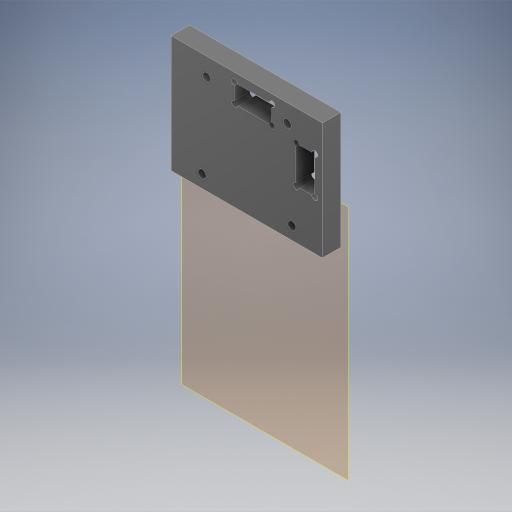
# Autodesk Inventor part: battery sideplate
Saved by Autodesk Inventor 2024 (Build 280153000, 153)
## iProperties
Created: 2024-09-04
Part Number: battery sideplate
Material: PMMA 플라스틱
Document SubType Name: Modeling
Designer: msi
Density: 1.188 g/cm^3
Appearance: 매끄러움 - 검은색
Author: msi
Autodesk Inventor part; units mm, degrees
ref_plane "YZ Plane" through (0, 0, 0) normal (1, 0, 0) x (0, 1, 0)
ref_plane "XZ Plane" through (0, 0, 0) normal (0, 1, 0) x (-1, 0, 0)
ref_plane "XY Plane" through (0, 0, 0) normal (0, 0, 1) x (1, 0, 0)
ref_plane "작업 평면1" through (0, 0, 0) normal (0, 0, 1) x (1, 0, 0)
sketch "스케치1" plane through (0, 0, 0) normal (0, 0, 1) x (1, 0, 0)
  line L0 (14.6, 27) -> (14.6, -35) projected
  line L1 (14.6, -35) -> (24.6, -35) projected
  line L2 (24.6, -35) -> (24.6, 35) projected
  line L3 (24.6, 35) -> (-24.6, 35) projected
  line L4 (-24.6, 35) -> (-24.6, -35) projected
  line L5 (-24.6, -35) -> (-14.6, -35) projected
  line L6 (-14.6, -35) -> (-14.6, 27) projected
  line L7 (-14.6, 27) -> (14.6, 27) projected
  circle A0 centre (-14.6, 30) radius 1.35 projected
  circle A1 centre (14.6, 30) radius 1.35 projected
  circle A2 centre (-17.3, -31) radius 1.35 projected
  circle A3 centre (-17.3, 13) radius 1.35 projected
  circle A4 centre (-17.3, -9) radius 1.35 projected
  circle A5 centre (17.3, -9) radius 1.35 projected
  circle A6 centre (17.3, 13) radius 1.35 projected
  circle A7 centre (17.3, -31) radius 1.35 projected
  line L8 (-24.6, 26) -> (24.6, 26)
  line L9 (24.6, 26) -> (24.6, 64)
  line L10 (-24.6, 64) -> (-24.6, 26)
  line L11 (22.1, 41.9) -> (16, 41.9)
  line L12 (16, 41.9) -> (16, 54)
  line L13 (16, 54) -> (22.1, 54)
  line L14 (22.1, 54) -> (22.1, 41.9)
  line L15 (8.1, 55) -> (-4, 55)
  line L16 (-4, 55) -> (-4, 61.1)
  line L17 (-4, 61.1) -> (8.1, 61.1)
  line L18 (8.1, 61.1) -> (8.1, 55)
  line L19 (-4, 64) -> (24.6, 64)
  line L20 (-24.6, 64) -> (-4, 64)
  point P0 (0, 0)
  dimension "d1" = 6.1
  dimension "d2" = 12.1
  dimension "d11" = 6.1
  constraints: 26 end point, 5 parallel, 4 perpendicular, 3 horizontal, 2 point on line, 1 collinear
  measures "d1" distance of L12.end L13.end
  measures "d2" distance of L11.end L12.end
  measures "d11" distance of L15.end L16.end
extrude "돌출2" add sketch "스케치1" along normal blind 6 contours L7 L6 L8 L4 L3 L2 L0 | L0 L8 L6 L7 | L3 L10 L20 L19 L9
sketch "스케치2" plane through (0, 0, 0) normal (0, 0, -1) x (-1, 0, 0)
  line L0 (-8.1, 61.1) -> (-8.1, 55) projected
  circle A0 centre (-13.1, 58) radius 1.35
  circle A1 centre (13.1, 58) radius 1.35
  point P0 (0, 0)
  dimension "d14" = 2.7
  dimension "d15" = 2.7
  constraints: 2 centre point
  measures "d14" diameter of A0
  measures "d15" diameter of A1
extrude "돌출3" cut sketch "스케치2" against normal through all
sketch "스케치3" plane through (0, 0, 6) normal (0, 0, 1) x (1, 0, 0)
  line L0 (8.1, 55) -> (-4, 55) projected
  line L1 (8.1, 61.1) -> (8.1, 55) projected
  line L2 (-4, 61.1) -> (8.1, 61.1) projected
  line L3 (-4, 55) -> (-4, 61.1) projected
  line L4 (16, 54) -> (22.1, 54) projected
  line L5 (22.1, 41.9) -> (16, 41.9) projected
  line L6 (22.1, 54) -> (22.1, 41.9) projected
  line L7 (16, 41.9) -> (16, 54) projected
  circle A0 centre (-4, 61.1) radius 1
  circle A1 centre (8.1, 61.1) radius 1
  circle A2 centre (8.1, 55) radius 1
  circle A3 centre (-4, 55) radius 1
  circle A4 centre (16, 54) radius 1
  circle A5 centre (22.1, 54) radius 1
  circle A6 centre (22.1, 41.9) radius 1
  circle A7 centre (16, 41.9) radius 1
  point P0 (0, 0)
  point P1 (22.1, 53)
  point P2 (21.1, 54)
  dimension "d18" = 2
  dimension "d19" = 2
  dimension "d20" = 2
  dimension "d21" = 2
  dimension "d22" = 2
  dimension "d23" = 2
  dimension "d24" = 2
  dimension "d25" = 2
  constraints: 8 centre point, 8 coincident
  measures "d18" diameter of A0
  measures "d19" diameter of A1
  measures "d20" diameter of A2
  measures "d21" diameter of A3
  measures "d22" diameter of A4
  measures "d23" diameter of A5
  measures "d24" diameter of A6
  measures "d25" diameter of A7
extrude "돌출4" cut sketch "스케치3" against normal blind 10 contours A3 L3 L0 | L0 L3 A3 | A2 L1 L0 | L0 L1 A2 | A0 L2 L3 | L3 L2 A0 | A1 L2 L1 | L1 L2 A1 | L7 A4 L4 | L4 A4 L7 | A5 L6 L4 | A7 L5 L7 | L7 L5 A7 | A6 L5 L6 | L6 L5 A6 picked at (21.7924, 54.586)
